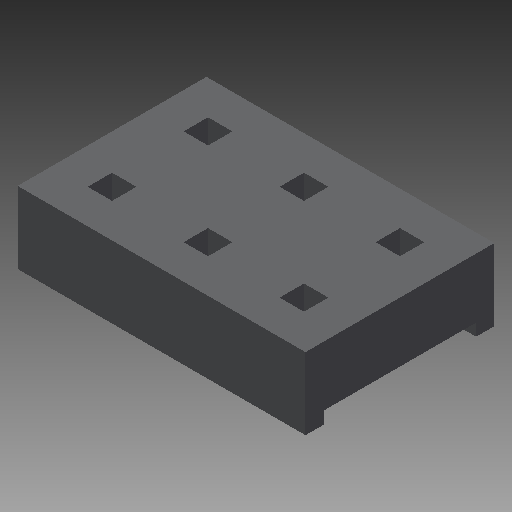
# Autodesk Inventor part: TMM-103-05-F-D_body
Saved by Autodesk Inventor 2019 (Build 230136000, 136)
## iProperties
Category: PARTsolutions
Company: SAMTEC
Created: 2019-03-13
Part Number: TMM-103-05-F-D_body
Material: Generico
Catalog Web Link: www.cadenas.de
Description: TMM Body-TMM Series
Vendor: SAMTEC
Document SubType Name: Modeling
Designer: psadmin
Manufacturer: SAMTEC
Mass: 0.028634 g
Surface Area: 0.905395 cm^2
Volume: 0.028634 cm^3
Density: 1 g/cm^3
Appearance: PSOLRGB-127-127-127
PSOL_IDENT_0: {$CADENAS_DATA\23d-libs\samtec\modelling\tmm\parts\tmm_body.prj},230 {VTYP=3D},{NB=TMM-103-05-F-D_bo
PSOL_IDENT_1: dy},{LINA=TMM-103-05-F-D_body},{NN=TMM Body},{DATE=15.05.2015 12:28:13},{GEOMDATE=12.11.2014 13:29:4
PSOL_IDENT_2: 7},{VERSION=},{LINEID=10},{WBVAR=POS,LS,PLOPT,ROW,TOPT,AOPT,RCOPT,POLOPT,KOPT,TROPT},{WBNUMERIC=}  {
PSOL_IDENT_3: NB=TMM-103-05-F-D_body},{LINA=TMM-103-05-F-D_body},{KT=DUMMY},{PN=TMM-103-05-F-D},{SERIES=TMM},{POS=
PSOL_IDENT_4: 03},{LS=05},{LEADSTALG=},{PLOPT=F},{PLOPTALG= '-L','10micro\" (0,25 microm) Gold on contact, Matte T
PSOL_IDENT_5: in on tail','-S','30micro\" (0,76 microm) Gold on contact, Matte Tin on tail' },{ROW=D},{ROWOPTALG= '
PSOL_IDENT_6: S','S:Single row','D','D:Double Row','Q','Q:Quad Row' },{TOPT=},{TOPTALG= '','Straight','-SM','SM: S
PSOL_IDENT_7: urface Mount' },{SH=160},{STACKERHALG=[120:323/5]},{TAILL=090},{TAILLALG='000','005','010','015','02
PSOL_IDENT_8: 0','025','030','035','040','045','050','055','060','065','070','075','080','085','090','095','100','
PSOL_IDENT_9: 105','110','115','120','125','130','135','140','145','150','155','160'},{AOPT=},{AOPTALG= '','Not Av
PSOL_IDENT_10: ailable' },{RCOPT=},{RCOPTALG= '','Not Available' },{POLOPT=Not Selected},{POLARIZEALG='001','002','
PSOL_IDENT_11: 003','004','005','006'},{POLARIZEPN=},{KOPT=},{KOPTALG= '','Not Available' },{TROPT=},{TROPTALG= '','
PSOL_IDENT_12: Not Available' },{L=0.23622},{W=0.155},{OAL=0.323},{STACKERHMAX=323},{POLMAX='001','002','003','004'
PSOL_IDENT_13: ,'005','006','007','008','009','010','011','012','013','014','015','016','017','018','019','020','02
PSOL_IDENT_14: 1','022','023','024','025','026','027','028','029','030','031','032','033','034','035','036','037','
PSOL_IDENT_15: 038','039','040','041','042','043','044','045','046','047','048','049','050','051','052','053','054'
PSOL_IDENT_16: ,'055','056','057','058','059','060','061','062','063','064','065','066','067','068','069','070','07
PSOL_IDENT_17: 1','072','073','074','075','076','077','078','079','080','081','082','083','084','085','086','087','
PSOL_IDENT_18: 088','089','090','091','092','093','094','095','096','097','098','099','100','101','102','103','104'
PSOL_IDENT_19: ,'105','106','107','108','109','110','111','112','113','114','115','116','117','118','119','120','12
PSOL_IDENT_20: 1','122','123','124','125','126','127','128','129','130','131','132','133','134','135','136','137','
PSOL_IDENT_21: 138','139','140','141','142','143','144','145','146','147','148','149','150','151','152','153','154'
PSOL_IDENT_22: ,'155','156','157','158','159','160','161','162','163','164','165','166','167','168','169','170','17
PSOL_IDENT_23: 1','172','173','174','175','176','177','178','179','180','181','182','183','184','185','186','187','
PSOL_IDENT_24: 188','189','190','191','192','193','194','195','196','197','198','199','200','201','202','203','204'
PSOL_IDENT_25: ,'205','206','207','208','209','210','211','212','213','214','215','216','217','218','219','220','22
PSOL_IDENT_26: 1','222','223','224','225','226','227','228','229','230','231','232','233','234','235','236','237','
PSOL_IDENT_27: 238','239','240','241','242','243','244','245','246','247','248','249','250','251','252','253','254'
PSOL_IDENT_28: ,'255','256','257','258','259','260','261','262','263','264','265','266','267','268','269','270','27
PSOL_IDENT_29: 1','272','273','274','275','276','277','278','279','280','281','282','283','284','285','286','287','
PSOL_IDENT_30: 288','289','290','291','292','293','294','295','296','297','298','299','300'},{TEST2='001','002','00
PSOL_IDENT_31: 3','004','005','006'},{TRUNC=6},{MIN=0.163},{PINSNUM=3},{POLLR=0},{TAILLMAX=163},{TAILLRANGE='000','
PSOL_IDENT_32: 005','010','015','020','025','030','035','040','045','050','055','060','065','070','075','080','085'
PSOL_IDENT_33: ,'090','095','100','105','110','115','120','125','130','135','140','145','150','155','160','165','17
PSOL_IDENT_34: 0','175','180','185','190','195','200','205','210','215','220','225','230','235','240','245','250','
PSOL_IDENT_35: 255','260','265','270','275','280','285','290','295','300','305','310','315','320','325','330','335'
PSOL_IDENT_36: ,'340','345','350','355','360','365','370','375','380','385','390','395','400','405','410','415','42
PSOL_IDENT_37: 0','425','430','435','440','445','450','455','460','465','470','475','480','485','490','495','500','
PSOL_IDENT_38: 505','510','515','520','525','530','535','540','545','550','555','560','565','570','575','580','585'
PSOL_IDENT_39: ,'590','595','600','605','610','615','620','625','630','635','640','645','650','655','660','665','67
PSOL_IDENT_40: 0','675','680','685','690','695','700','705','710','715','720','725','730','735','740','745','750','
PSOL_IDENT_41: 755','760','765','770','775','780','785','790','795','800','805','810','815','820','825','830','835'
PSOL_IDENT_42: ,'840','845','850','855','860','865','870','875','880','885','890','895','900','905','910','915','92
PSOL_IDENT_43: 0','925','930','935','940','945','950','955','960','965','970','975','980','985','990','995'},{TAILL
PSOL_IDENT_44: TRUNC=33},{TAILLNUM=0.09},{ROWNO=2},{POLPLANEPOS=0},{POLPINPOS=0},{TOPCUT=0.198}
NN: TMM Body
NT: TMM Series
NB: TMM-103-05-F-D_body
NBSYN: $PN._body
LINA: TMM-103-05-F-D_body
SERIES: TMM
POS: 03
LS: 05
PLOPT: -F: 3u" Selective Gold on Contact, Matte Tin on Tail
ROW: D:Double Row
TOPT: Straight
SH: 160
AOPT: Not Available
RCOPT: Not Available
POLOPT: Not Selected
KOPT: Not Available
TROPT: Not Available
POLMAX: '001','002','003','004','005','006','007','008','009','010','011','012','013','014','015','016','017','018','019','020','021','022','023','024','025','026','027','028','029','030','031','032','033','034','035','036','037','038','039','040','041','042','043','044','045','046','047','048','049','050','051','052','053','054','055','056','057','058','059','060','061','062','063','064','065','066','067','068','069','070','071','072','073','074','075','076','077','078','079','080','081','082','083','084','085','086','087','088','089','090','091','092','093','094','095','096','097','098','099','100','101','102','103','104','105','106','107','108','109','110','111','112','113','114','115','116','117','118','119','120','121','122','123','124','125','126','127','128','129','130','131','132','133','134','135','136','137','138','139','140','141','142','143','144','145','146','147','148','149','150','151','152','153','154','155','156','157','158','159','160','161','162','163','164','165','166','167','168','169','170','171','172','173','174','175','176','177','178','179','180','181','182','183','184','185','186','187','188','189','190','191','192','193','194','195','196','197','198','199','200','201','202','203','204','205','206','207','208','209','210','211','212','213','214','215','216','217','218','219','220','221','222','223','224','225','226','227','228','229','230','231','232','233','234','235','236','237','238','239','240','241','242','243','244','245','246','247','248','249','250','251','252','253','254','255','256','257','258','259','260','261','262','263','264','265','266','267','268','269','270','271','272','273','274','275','276','277','278','279','280','281','282','283','284','285','286','287','288','289','290','291','292','293','294','295','296','297','298','299','300'
TAILLRANGE: '000','005','010','015','020','025','030','035','040','045','050','055','060','065','070','075','080','085','090','095','100','105','110','115','120','125','130','135','140','145','150','155','160','165','170','175','180','185','190','195','200','205','210','215','220','225','230','235','240','245','250','255','260','265','270','275','280','285','290','295','300','305','310','315','320','325','330','335','340','345','350','355','360','365','370','375','380','385','390','395','400','405','410','415','420','425','430','435','440','445','450','455','460','465','470','475','480','485','490','495','500','505','510','515','520','525','530','535','540','545','550','555','560','565','570','575','580','585','590','595','600','605','610','615','620','625','630','635','640','645','650','655','660','665','670','675','680','685','690','695','700','705','710','715','720','725','730','735','740','745','750','755','760','765','770','775','780','785','790','795','800','805','810','815','820','825','830','835','840','845','850','855','860','865','870','875','880','885','890','895','900','905','910','915','920','925','930','935','940','945','950','955','960','965','970','975','980','985','990','995'
SUPPLIER: SAMTEC
ARTICLENO: TMM-103-05-F-D_body
BOMINFO: TMM-103-05-F-D_body
CREATOR: CADENAS GmbH
Title: TMM-103-05-F-D_body
Author: Cadenas PARTsolutions
Comments: TMM Series
Autodesk Inventor part; units mm, degrees
ref_plane "YZ Plane" through (0, 0, 0) normal (1, 0, 0) x (0, 1, 0)
ref_plane "XZ Plane" through (0, 0, 0) normal (0, 1, 0) x (-1, 0, 0)
ref_plane "XY Plane" through (0, 0, 0) normal (0, 0, 1) x (1, 0, 0)
sketch "Sketch0" plane through (0, 0, 0) normal (0, 1, 0) x (1, 0, 0)
  line L0 (-3, -1.9685) -> (3, -1.9685)
  line L1 (3, -1.9685) -> (3, 1.9685)
  line L2 (3, 1.9685) -> (-3, 1.9685)
  line L3 (-3, 1.9685) -> (-3, -1.9685)
  line L4 (1.746, 0.746) -> (2.254, 0.746)
  line L5 (2.254, 0.746) -> (2.254, 1.254)
  line L6 (2.254, 1.254) -> (1.746, 1.254)
  line L7 (1.746, 1.254) -> (1.746, 0.746)
  line L8 (1.746, -1.254) -> (2.254, -1.254)
  line L9 (2.254, -1.254) -> (2.254, -0.746)
  line L10 (2.254, -0.746) -> (1.746, -0.746)
  line L11 (1.746, -0.746) -> (1.746, -1.254)
  line L12 (-0.254, 0.746) -> (0.254, 0.746)
  line L13 (0.254, 0.746) -> (0.254, 1.254)
  line L14 (0.254, 1.254) -> (-0.254, 1.254)
  line L15 (-0.254, 1.254) -> (-0.254, 0.746)
  line L16 (-0.254, -1.254) -> (0.254, -1.254)
  line L17 (0.254, -1.254) -> (0.254, -0.746)
  line L18 (0.254, -0.746) -> (-0.254, -0.746)
  line L19 (-0.254, -0.746) -> (-0.254, -1.254)
  line L20 (-2.254, 0.746) -> (-1.746, 0.746)
  line L21 (-1.746, 0.746) -> (-1.746, 1.254)
  line L22 (-1.746, 1.254) -> (-2.254, 1.254)
  line L23 (-2.254, 1.254) -> (-2.254, 0.746)
  line L24 (-2.254, -1.254) -> (-1.746, -1.254)
  line L25 (-1.746, -1.254) -> (-1.746, -0.746)
  line L26 (-1.746, -0.746) -> (-2.254, -0.746)
  line L27 (-2.254, -0.746) -> (-2.254, -1.254)
  constraints: 56 end point
extrude "Extrusion1" add sketch "Sketch0" along normal blind 1.4986
sketch "Sketch1" plane through (3, 0, 0) normal (1, 0, 0) x (0, 0, -1)
  line L0 (-1.5875, 0.254) -> (-1.5875, 0)
  line L1 (-1.5875, 0) -> (1.5875, 0)
  line L2 (1.5875, 0) -> (1.5875, 0.254)
  line L3 (1.5875, 0.254) -> (-1.5875, 0.254)
  constraints: 8 end point
extrude "Extrusion2" cut sketch "Sketch1" against normal blind 6
ref_plane "0_XY" through (0, 0, 0) normal (0, 1, 0) x (1, 0, 0)
ref_plane "0_YZ" through (0, 0, 0) normal (1, 0, 0) x (0, 0, -1)
ref_plane "0_ZX" through (0, 0, 0) normal (0, 0, -1) x (0, 1, 0)
body "Solid1"
